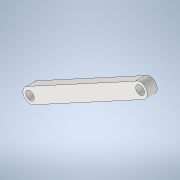
# Autodesk Inventor part: Palanca_metacarpo_proxima
Saved by Autodesk Inventor 2020.4 (Build 244396010, 396A)
## iProperties
Created: 2021-11-11
Part Number: Palanca_metacarpo_proxima
Material: Generic
Document SubType Name: Modeling
Designer: chalo
Density: 1 g/cm^3
Appearance: Default
Author: chalo
Autodesk Inventor part; units mm, degrees
ref_plane "YZ Plane" through (0, 0, 0) normal (1, 0, 0) x (0, 1, 0)
ref_plane "XZ Plane" through (0, 0, 0) normal (0, 1, 0) x (-1, 0, 0)
ref_plane "XY Plane" through (0, 0, 0) normal (0, 0, 1) x (1, 0, 0)
sketch "Sketch1" plane through (0, 0, 0) normal (0, 0, 1) x (1, 0, 0)
  circle A0 centre (3.75, -3.0891) radius 1.55 projected
  circle A1 centre (43.2497, 18.3605) radius 1.6 projected
  circle A2 centre (3.75, -3.0891) radius 2.55
  circle A3 centre (43.2497, 18.3605) radius 2.6
  line L0 (2.5356, -0.8468) -> (41.4312, 20.2187)
  line L1 (44.4879, 16.0743) -> (4.9644, -5.3314)
  point P0 (0, 0)
  dimension "d0" = 1
  dimension "d1" = 1
  constraints: 4 end point, 4 point on circle, 3 tangent, 2 centre point, 1 parallel
  measures "d0" radial gap between concentric circles of A0 A2
  measures "d1" radial gap between concentric circles of A1 A3
extrude "Extrusion1" add sketch "Sketch1" along normal mid plane 3.5
body "Solid1"
